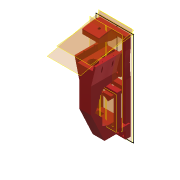
# Autodesk Inventor part: 08_Opentrons_Autofocus_flexurebaering
Saved by Autodesk Inventor 2019.4 (Build 234330000, 330)
## iProperties
Created: 2020-11-20
Part Number: 08_Opentrons_Autofocus_flexurebaering
Material: Generic
Document SubType Name: Modeling
Designer: diederichbenedict
Density: 1 g/cm^3
Appearance: Light Red
Author: diederichbenedict
Autodesk Inventor part; units mm, degrees
ref_plane "YZ Plane" through (0, 0, 0) normal (1, 0, 0) x (0, 1, 0)
ref_plane "XZ Plane" through (0, 0, 0) normal (0, 1, 0) x (-1, 0, 0)
ref_plane "XY Plane" through (0, 0, 0) normal (0, 0, 1) x (1, 0, 0)
ref_plane "Work Plane1" through (0, 0, 0) normal (0, 0, 1) x (1, 0, 0)
sketch "Sketch1" plane through (0, 0, 0) normal (0, 0, 1) x (1, 0, 0)
  line L0 (17.158547, 59.978654) -> (2.158547, 59.978654) construction
  line L1 (2.158547, 59.978654) -> (2.158547, 62.700785) construction
  line L2 (2.158547, 62.700785) -> (17.158547, 62.700785) construction
  line L3 (17.158547, 62.700785) -> (17.158547, 91.339719) construction
  line L4 (6.864659, 91.339719) -> (-18.841453, 91.339719) construction
  line L5 (-18.841453, 91.339719) -> (-18.841453, -14.660281) construction
  line L6 (-18.841453, -14.660281) -> (17.158547, -14.660281) construction
  line L7 (17.158547, -14.660281) -> (17.158547, 59.978654) construction
  line L8 (13.858547, 17.339719) -> (13.863005, 4.639719) construction
  line L9 (13.863005, 4.639719) -> (6.678294, 4.639719) construction
  arc A0 (-15.691453, 17.339719) -> (6.678294, 4.639719) centre (-0.935341, 17.280089) ccw construction
  arc A1 (6.678294, 30.039719) -> (-15.691453, 17.339719) centre (-0.935341, 17.399349) ccw construction
  line L10 (13.863005, 30.039719) -> (6.678294, 30.039719) construction
  line L11 (13.858547, 17.339719) -> (13.863005, 30.039719) construction
  circle A2 centre (-0.935341, 17.399349) radius 10.125
  line L12 (17.158547, -14.660281) -> (-0.935341, -14.660281)
  line L13 (-0.935341, -14.660281) -> (-0.935341, -0.660281)
  line L14 (-0.935341, -0.660281) -> (17.158547, -0.660281)
  line L15 (17.158547, -0.660281) -> (17.158547, -14.660281)
  line L16 (17.158547, 0.876503) -> (13.158547, 0.876503)
  line L17 (13.158547, 0.876503) -> (13.158547, 91.339719)
  line L18 (13.158547, 91.339719) -> (17.158547, 91.339719)
  line L19 (13.158547, 34.280089) -> (-0.935341, 34.280089)
  line L20 (-0.935341, 34.280089) -> (-0.935341, 38.280089)
  line L21 (-0.935341, 38.280089) -> (13.158547, 38.280089)
  line L22 (13.158547, 38.280089) -> (13.158547, 34.280089)
  line L23 (13.158547, 91.339719) -> (-0.935341, 91.339719)
  line L24 (-0.935341, 91.339719) -> (-0.935341, 86.339719)
  line L25 (-0.935341, 86.339719) -> (13.158547, 86.339719)
  line L26 (13.158547, 86.339719) -> (13.158547, 91.339719)
  line L27 (-0.935341, 91.339719) -> (2.064659, 91.339719)
  line L28 (2.064659, 91.339719) -> (2.064659, 103.339719)
  line L29 (2.064659, 103.339719) -> (-0.935341, 103.339719)
  line L30 (-0.935341, 103.339719) -> (-0.935341, 91.339719)
  arc A3 (-5.635247, 28.982133) -> (3.120733, 29.222981) centre (-0.935341, 17.399349) ccw
  arc A4 (-5.635247, 28.982133) -> (3.120733, 29.222981) centre (-0.935341, 17.399349) ccw
  line L31 (14.111603, -3.660281) -> (2.111603, -3.660281) construction
  line L32 (2.111603, -3.660281) -> (2.111603, -11.660281) construction
  line L33 (2.111603, -11.660281) -> (14.111603, -11.660281) construction
  line L34 (14.111603, -11.660281) -> (14.111603, -3.660281) construction
  line L35 (14.111603, -3.660281) -> (2.111603, -11.660281) construction
  line L36 (2.111603, -3.660281) -> (14.111603, -11.660281) construction
  circle A5 centre (14.111603, -3.660281) radius 1.45
  circle A6 centre (14.111603, -11.660281) radius 1.45
  circle A7 centre (2.111603, -3.660281) radius 1.45
  circle A8 centre (2.111603, -11.660281) radius 1.45
  circle A9 centre (-0.935341, 17.399349) radius 10.125
  circle A10 centre (7.722275, -11.660281) radius 1.45
  circle A11 centre (7.722275, -3.660281) radius 1.45
  circle A12 centre (-8.847508, 49.748913) radius 1.45
  circle A13 centre (-9.592957, -3.660281) radius 1.45
  circle A14 centre (7.722275, -3.660281) radius 1.45
  circle A15 centre (14.111603, -11.660281) radius 1.45
  circle A16 centre (7.722275, -11.660281) radius 1.45
  circle A17 centre (-9.592957, -11.660281) radius 1.45
  circle A18 centre (-15.982285, -11.660281) radius 1.45
  circle A19 centre (6.976826, 49.748913) radius 1.45
  line L37 (17.158547, 91.339719) -> (6.864659, 91.339719)
  arc A20 (17.158547, 76.029134) -> (17.158547, 46.231552) centre (138.700705, 61.130343) ccw
  line L38 (17.158547, 91.339719) -> (17.158547, 76.029134)
  line L39 (17.158547, 46.231552) -> (17.158547, 0.876503)
  point P0 (8.111603, -7.660281)
  dimension "d19" = 14
  dimension "d20" = 4
  dimension "d21" = 4
  dimension "d37" = 5
  dimension "d38" = 3
  dimension "d39" = 12
  dimension "d41" = 17
  dimension "d60" = 0
  dimension "d61" = 0
  dimension "d62" = 0
  dimension "d63" = 12
  dimension "d64" = 8
  dimension "d65" = 2.9
  dimension "d66" = 2.9
  dimension "d67" = 2.9
  dimension "d68" = 2.9
  dimension "d83" = 2.9
  dimension "d84" = 2.9
  constraints: 55 end point, 13 parallel, 7 centre point, 6 horizontal, 6 perpendicular, 6 point on line, 4 coincident, 2 midpoint, 2 point on circle
  measures "d19" distance of L12.end L13.end
  measures "d20" distance of L17.end L18.end
  measures "d21" distance of L19.end L20.end
  measures "d37" distance of L24.end L23.end
  measures "d38" distance of L29.end L28.end
  measures "d39" distance of L28.end L27.end
  measures "d41" distance from line of L19 A0.centre
  measures "d60" distance from line of L13 A0.centre
  measures "d61" distance from line of A0.centre L20
  measures "d62" distance from line of A1.centre L24
  measures "d63" distance of L33.end L32.end
  measures "d64" distance of L32.end L31.end
  measures "d65" diameter of A5
  measures "d66" diameter of A6
  measures "d67" diameter of A7
  measures "d68" diameter of A8
  measures "d83" diameter of A10
  measures "d84" diameter of A11
extrude "Extrusion1" add sketch "Sketch1" along normal blind 6 contours L12 L13 L14 L15 | L16 L17 L18 L38 A20 L39 | L19 L20 L21 L17 | L25 L24 L23 L17 | A5 | A7 | A8
ref_plane "Work Plane2" through (0, 0, 11) normal (0, 0, 1) x (1, 0, 0)
sketch "Sketch2" plane through (0, 0, 11) normal (0, 0, 1) x (1, 0, 0)
  line L0 (-0.935341, 34.280089) -> (13.158547, 34.280089)
  line L1 (13.158547, 34.280089) -> (13.158547, 0.876503)
  line L2 (13.158547, 0.876503) -> (17.158547, 0.876503)
  line L3 (17.158547, 76.029134) -> (17.158547, 91.339719) construction
  line L4 (17.158547, 91.339719) -> (-0.935341, 91.339719) construction
  line L5 (13.158547, 86.339719) -> (13.158547, 38.280089) construction
  line L6 (13.158547, 38.280089) -> (-0.935341, 38.280089)
  line L7 (-0.935341, 38.280089) -> (-0.935341, 34.280089)
  line L8 (13.158547, 38.280089) -> (-0.935341, 38.280089)
  line L9 (13.158547, 38.280089) -> (17.158547, 38.280089)
  line L10 (17.158547, 91.339719) -> (-0.935341, 91.339719) construction
  line L11 (13.158547, 91.339719) -> (-0.935341, 91.339719) construction
  line L12 (-0.935341, 91.339719) -> (-0.935341, 86.339719) construction
  line L13 (-0.935341, 86.339719) -> (13.158547, 86.339719) construction
  line L14 (13.158547, 86.339719) -> (13.158547, 91.339719) construction
  line L15 (-0.935341, 91.339719) -> (2.064659, 91.339719) construction
  line L16 (2.064659, 91.339719) -> (2.064659, 99.339719) construction
  line L17 (2.064659, 99.339719) -> (-0.935341, 99.339719) construction
  line L18 (-0.935341, 99.339719) -> (-0.935341, 91.339719) construction
  line L19 (-0.935341, 91.339719) -> (-0.935341, 86.339719) construction
  line L20 (-0.935341, 86.339719) -> (13.158547, 86.339719) construction
  line L21 (17.158547, 0.876503) -> (17.158547, 46.231552)
  arc A0 (17.158547, 76.029134) -> (17.158547, 46.231552) centre (138.700705, 61.130343) ccw construction
  line L22 (-0.935341, 38.280089) -> (13.158547, 38.280089)
  line L23 (-0.935341, 38.280089) -> (17.158547, 38.280089)
  line L24 (17.158547, 38.280089) -> (17.158547, 34.280089)
  line L25 (17.158547, 34.280089) -> (-0.935341, 34.280089)
  line L26 (-0.935341, 34.280089) -> (-0.935341, 38.280089)
  line L27 (13.158547, 0.876503) -> (17.158547, 0.876503)
  line L28 (17.158547, 34.280089) -> (13.158547, 34.280089)
  line L29 (13.158547, 34.280089) -> (13.158547, 0.876503)
  line L30 (13.158547, 0.876503) -> (17.158547, 0.876503)
  line L31 (17.158547, 0.876503) -> (17.158547, 34.280089)
  point P0 (0, 0)
  point P1 (2.064659, 91.339719)
  dimension "d34" = 5
  dimension "d35" = 3
  dimension "d36" = 8
  constraints: 34 end point, 8 parallel, 5 perpendicular, 4 horizontal, 2 point on line
  measures "d34" distance of L12.end L10.end
  measures "d35" distance of L17.end L16.end
  measures "d36" distance of L16.end L15.end
extrude "Extrusion2" add sketch "Sketch2" along normal blind 5
sketch "Sketch3" plane through (17.158547, -14.660281, 0) normal (1, 0, 0) x (0, 0, -1)
  line L0 (0, 14) -> (0, 0)
  line L1 (0, 14) -> (-6, 14)
  line L2 (-6, 0) -> (-6, 14)
  line L3 (0, 0) -> (-6, 0)
  line L4 (0, 90.689414) -> (0, 106)
  line L5 (0, 106) -> (-6, 106)
  line L6 (-6, 90.689414) -> (-6, 106)
  line L7 (-11, 106) -> (-11, 94.797626)
  line L8 (-16, 94.797626) -> (-16, 106)
  line L9 (-6, 14) -> (-6, 0)
  line L10 (-11.5, 14.036784) -> (-6, 14.036784)
  line L11 (-6, 14.036784) -> (-6, 9.036784)
  line L12 (-6, 9.036784) -> (-11.5, 9.036784)
  line L13 (-11.5, 9.036784) -> (-11.5, 14.036784)
  line L14 (-11, 15.536784) -> (-16, 15.536784)
  line L15 (-11, 15.536784) -> (-11.5, 15.536784)
  line L16 (-11.5, 15.536784) -> (-11.5, 14.036784)
  line L17 (-11.5, 14.036784) -> (-11, 14.036784)
  line L18 (-11, 14.036784) -> (-11, 15.536784)
  line L19 (0, 15.536784) -> (-0.5, 15.536784)
  line L20 (-0.5, 15.536784) -> (-0.5, 14)
  line L21 (-0.5, 14) -> (0, 14)
  line L22 (0, 14) -> (0, 15.536784)
  line L23 (-6, 15.536784) -> (-6, 106)
  line L24 (-6, 54.44037) -> (-11.5, 54.44037)
  line L25 (-11.5, 54.44037) -> (-11.5, 59.44037)
  line L26 (-11.5, 59.44037) -> (-6, 59.44037)
  line L27 (-6, 59.44037) -> (-6, 54.44037)
  line L28 (-11, 52.94037) -> (-16, 52.94037)
  line L29 (-11, 52.94037) -> (-11.5, 52.94037)
  line L30 (-11.5, 52.94037) -> (-11.5, 54.44037)
  line L31 (-11.5, 54.44037) -> (-11, 54.44037)
  line L32 (-11, 54.44037) -> (-11, 52.94037)
  line L33 (0, 90.689414) -> (-6, 90.689414)
  line L34 (-11, 106) -> (-16, 106)
  line L35 (-11, 94.797626) -> (-16, 94.797626)
  point P0 (0, 14.660281)
  dimension "d25" = 5
  dimension "d26" = 0.5
  dimension "d27" = 0.5
  dimension "d28" = 5
  dimension "d29" = 0.5
  dimension "d40" = 0
  constraints: 40 end point, 10 parallel, 6 point on line, 5 horizontal, 5 perpendicular
  measures "d25" distance of L10.end L11.end
  measures "d26" distance of L17.end L16.end
  measures "d27" distance of L21.end L20.end
  measures "d28" distance of L24.end L25.end
  measures "d29" distance of L30.end L31.end
  measures "d40" distance between parallel lines of L30 L25
extrude "Extrusion3" add sketch "Sketch3" against normal up to surface (4 mm away) contours L1 L20 L19 L22 | L2 L12 L13 L10 L11 | L10 L16 L14 L18
ref_plane "Work Plane3" through (0, 0, 18) normal (0, 0, 1) x (1, 0, 0)
sketch "Sketch4" plane through (0, 0, 18) normal (0, 0, 1) x (1, 0, 0)
  line L0 (17.158547, 34.889127) -> (-18.841453, 34.889127)
  line L1 (-0.935341, 34.280089) -> (13.158547, 34.280089)
  line L2 (13.158547, 34.280089) -> (13.158547, 0.876503)
  line L3 (13.158547, 0.876503) -> (17.158547, 0.876503)
  line L4 (-0.935341, 38.280089) -> (-0.935341, 34.280089)
  line L5 (-4.526541, 27.364099) -> (2.655859, 27.364099)
  arc A0 (9.489986, 15.527045) -> (2.655859, 27.364099) centre (-0.935341, 17.399349) ccw
  line L6 (9.489986, 15.527045) -> (5.898786, 9.306903)
  arc A1 (-7.769468, 9.306903) -> (5.898786, 9.306903) centre (-0.935341, 17.399349) ccw
  line L7 (-7.769468, 9.306903) -> (-11.360668, 15.527045)
  arc A2 (-4.526541, 27.364099) -> (-11.360668, 15.527045) centre (-0.935341, 17.399349) ccw
  arc A3 (-3.214574, 30.399349) -> (-4.800903, 29.617364) centre (-3.214574, 28.399349) ccw
  arc A4 (-5.635247, 28.982133) -> (-4.800903, 29.617364) centre (-6.387232, 30.835378) ccw
  arc A5 (-5.635247, 28.982133) -> (3.120733, 29.222981) centre (-0.935341, 17.399349) ccw
  arc A6 (2.301156, 29.757056) -> (3.120733, 29.222981) centre (3.769704, 31.114762) ccw
  arc A7 (2.301156, 29.757056) -> (0.832608, 30.399349) centre (0.832608, 28.399349) ccw
  line L8 (0.832608, 30.399349) -> (-3.214574, 30.399349)
  arc A8 (2.411297, 29.858883) -> (0.832608, 30.549349) centre (0.832608, 28.399349) ccw
  arc A9 (2.411297, 29.858883) -> (3.169405, 29.364864) centre (3.769704, 31.114762) ccw
  arc A10 (-5.691646, 29.121126) -> (3.169405, 29.364864) centre (-0.935341, 17.399349) ccw
  arc A11 (-5.691646, 29.121126) -> (-4.919877, 29.708715) centre (-6.387232, 30.835378) ccw
  arc A12 (-3.214574, 30.549349) -> (-4.919877, 29.708715) centre (-3.214574, 28.399349) ccw
  line L9 (-3.214574, 30.549349) -> (0.832608, 30.549349)
  line L10 (8.265033, 26.081262) -> (11.868953, 29.685181)
  line L11 (8.265033, 26.081262) -> (13.361745, 26.081262) construction
  line L12 (11.868953, 29.685181) -> (11.868953, 32.780089)
  line L13 (11.868953, 32.780089) -> (-0.935341, 32.780089)
  line L14 (-0.935341, 38.280089) -> (-0.935341, 34.280089)
  line L15 (-0.935341, 33.557251) -> (-0.935341, 30.549349)
  line L16 (-0.935341, 32.780089) -> (-0.935341, 30.549349)
  line L17 (17.158547, 0.876503) -> (17.158547, 38.280089) construction
  line L18 (17.158547, 0.876503) -> (17.158547, 38.280089)
  line L19 (17.158547, 0.876503) -> (17.158547, 34.889127)
  line L20 (17.158547, 38.280089) -> (-0.935341, 38.280089)
  point P0 (0, 0)
  point P1 (17.158547, 49.748913)
  dimension "d43" = 0.15
  dimension "d44" = 45
  dimension "d49" = 1.5
  constraints: 18 end point, 11 point on circle, 5 centre point, 4 point on line, 2 horizontal, 2 vertical, 1 collinear, 1 equal length, 1 perpendicular, 7 other
  measures "d43" radial gap between concentric circles of A7 A8
  measures "d44" angle of L11 L10
  measures "d49" distance between parallel lines of L1 L13
extrude "Extrusion4" add sketch "Sketch4" against normal up to surface (18 mm away) contours A8 L9 L15 L13 L12 L10 A10 A9
sketch "Sketch5" plane through (-0.935341, 30.549349, 18) normal (-1, 0, 0) x (0, 0, 1)
  line L0 (-7, 3.73074) -> (-7, 7.73074)
  line L1 (-7, 3.73074) -> (-2, 3.73074)
  line L2 (-2, 7.73074) -> (-2, 3.73074)
  line L3 (-7, 7.73074) -> (-2, 7.73074)
  line L4 (-18, 0) -> (-18, 2.23074)
  line L5 (0, 0) -> (-18, 0)
  line L6 (0, 2.23074) -> (0, 0)
  line L7 (0, 2.23074) -> (-18, 2.23074)
  line L8 (-18, 3.73074) -> (-18, 7.73074)
  line L9 (-18, 3.73074) -> (-12, 3.73074)
  line L10 (-12, 7.73074) -> (-12, 3.73074)
  line L11 (-18, 7.73074) -> (-12, 7.73074)
  line L12 (0, 2.23074) -> (-18, 2.23074)
  line L13 (-18, 3.73074) -> (-17.5, 3.73074)
  line L14 (-17.5, 3.73074) -> (-17.5, 2.23074)
  line L15 (-17.5, 2.23074) -> (-18, 2.23074)
  line L16 (-18, 2.23074) -> (-18, 3.73074)
  line L17 (-7, 3.73074) -> (-6.5, 3.73074)
  line L18 (-6.5, 3.73074) -> (-6.5, 2.23074)
  line L19 (-6.5, 2.23074) -> (-7, 2.23074)
  line L20 (-7, 2.23074) -> (-7, 3.73074)
  point P0 (-18, -30.549349)
  dimension "d47" = 0.5
  dimension "d48" = 0.5
  constraints: 16 end point, 4 parallel, 2 horizontal, 2 perpendicular, 2 point on line
  measures "d47" distance of L14.end L15.end
  measures "d48" distance of L18.end L19.end
sketch "Sketch7" plane through (-0.935341, 32.780089, 18) normal (0, 1, 0) x (1, 0, 0)
  circle A0 centre (-0.255642, 2.740799) radius 1.45
  line L0 (-0.255642, 2.740799) -> (-0.255642, 18) construction
  line L1 (1.394358, 2.740799) -> (1.394358, 18)
  line L2 (-1.905642, 18) -> (-1.905642, 2.740799)
  arc A1 (-1.905642, 2.740799) -> (1.394358, 2.740799) centre (-0.255642, 2.740799) ccw
  arc A2 (1.394358, 18) -> (-1.905642, 18) centre (-0.255642, 18) ccw
  line L3 (-0.255642, 2.740799) -> (15.003559, 2.740799) construction
  point P0 (0.935341, 18)
  point P1 (-0.255642, 10.370399)
  dimension "d50" = 90
  dimension "d51" = 0.2
  constraints: 10 end point, 4 point on circle, 4 tangent, 2 centre point, 1 horizontal, 1 midpoint, 1 parallel, 1 perpendicular
  measures "d50" angle of L3 L0
  measures "d51" radial gap between concentric circles of A0 A1
extrude "Extrusion5" cut sketch "Sketch7" against normal blind 5 contours A0 | A1 L2 A2 L1
extrude "Extrusion6" add sketch "Sketch5" against normal up to surface (12.804294 mm away) contours L1 L18 L7 L20 | L7 L16 L9 L14
sketch "Sketch8" plane through (0, 0, 18) normal (0, 0, 1) x (1, 0, 0)
  arc A0 (2.411297, 29.858883) -> (0.832608, 30.549349) centre (0.832608, 28.399349) ccw
  arc A1 (2.411297, 29.858883) -> (3.169405, 29.364864) centre (3.769704, 31.114762) ccw
  arc A2 (8.265033, 26.081262) -> (3.169405, 29.364864) centre (-0.935341, 17.399349) ccw
  line L0 (8.265033, 26.081262) -> (11.868953, 29.685181)
  line L1 (11.868953, 29.685181) -> (11.868953, 32.780089)
  line L2 (11.868953, 32.780089) -> (-0.935341, 32.780089)
  line L3 (-0.935341, 32.780089) -> (-0.935341, 30.549349)
  line L4 (-0.935341, 30.549349) -> (0.832608, 30.549349)
  line L5 (11.868953, 34.280089) -> (11.868953, 32.780089)
  line L6 (-0.935341, 34.280089) -> (11.868953, 34.280089)
  line L7 (-0.935341, 32.780089) -> (-0.935341, 34.280089)
  line L8 (-0.935341, 32.780089) -> (0.459017, 32.780089)
  line L9 (11.868953, 32.780089) -> (0.459017, 32.780089)
  line L10 (-0.895411, 34.280089) -> (2.604589, 34.280089)
  line L11 (2.604589, 34.280089) -> (2.604589, 31.780089)
  line L12 (2.604589, 31.780089) -> (-0.895411, 31.780089)
  line L13 (-0.895411, 31.780089) -> (-0.895411, 34.280089)
  point P0 (0, 0)
  dimension "d56" = 3.5
  dimension "d57" = 2.5
  constraints: 8 end point, 2 parallel, 1 horizontal, 1 perpendicular, 1 point on line
  measures "d56" distance of L11.end L12.end
  measures "d57" distance of L10.end L11.end
extrude "Extrusion7" cut sketch "Sketch8" against normal through all contours L13 L6 L11 L2 | L2 L11 L12 L13
sketch "Sketch9" plane through (-0.935341, -14.660281, 0) normal (-1, 0, 0) x (0, 0, 1)
  line L0 (0, 0) -> (0, 14)
  line L1 (0, 0) -> (6, 0)
  line L2 (6, 14) -> (6, 0)
  line L3 (0, 14) -> (6, 14)
  line L4 (24.051888, 27.109882) -> (31.122956, 34.18095)
  line L5 (29.708742, 35.595164) -> (22.637674, 28.524096)
  line L6 (31.122956, 34.18095) -> (29.708742, 35.595164)
  line L7 (24.051888, 27.109882) -> (22.637674, 28.524096)
  line L8 (29.708742, 35.736585) -> (22.496253, 28.524096)
  line L9 (24.051888, 26.968461) -> (31.264377, 34.18095)
  line L10 (31.264377, 34.18095) -> (29.708742, 35.736585)
  line L11 (22.496253, 28.524096) -> (38.52182, 28.524096) construction
  line L12 (0, 14) -> (6, 14)
  line L13 (15.723556, 14) -> (6, 14)
  line L14 (6, 14) -> (6, 0)
  line L15 (29.708742, 35.736585) -> (29.708742, 57.736585)
  line L16 (29.708742, 57.736585) -> (0, 57.736585)
  line L17 (0, 101) -> (0, 52.94037)
  line L18 (0, 57.736585) -> (0, 63.736585)
  line L19 (0, 63.736585) -> (35.708742, 63.736585)
  line L20 (35.708742, 63.736585) -> (35.708742, 34.18095)
  line L21 (35.708742, 34.18095) -> (19.769903, 0)
  line L22 (0, 0) -> (6, 0)
  line L23 (19.769903, 0) -> (6, 0)
  line L24 (0, 57.736585) -> (22.116428, 54.292028)
  line L25 (22.116428, 54.292028) -> (29.708742, 35.736585)
  line L26 (15.723556, 14) -> (22.496253, 16.430232)
  line L27 (22.496253, 16.430232) -> (22.496253, 25.412826)
  line L28 (22.496253, 28.524096) -> (22.372688, 28.259109)
  line L29 (19.901381, 22.959376) -> (19.777816, 22.694389)
  line L30 (24.051888, 26.968461) -> (22.496253, 25.412826)
  line L31 (22.496253, 28.524096) -> (22.566964, 28.453385)
  line L32 (23.981177, 27.039172) -> (24.051888, 26.968461)
  point P0 (0, 14.660281)
  dimension "d69" = 0.1
  dimension "d71" = 22
  dimension "d72" = 6
  dimension "d73" = 6
  constraints: 48 end point, 7 point on line, 4 perpendicular, 3 parallel, 2 vertical, 1 collinear, 1 horizontal, 3 other
  measures "d69" distance between parallel lines of L6 L10
  measures "d71" distance of L8.start L15.end
  measures "d72" distance of L16.end L18.end
  measures "d73" distance between parallel lines of L20 L15
extrude "Extrusion8" add sketch "Sketch9" against normal blind 7 contours L2 L13 L26 L27 L30 L9 L10 L15 L16 L17 L19 L20 L21 L23 | L16 L15 L25 L24
sketch "Sketch10" plane through (-0.935341, 19.520669, 35.708742) normal (0, 0, 1) x (1, 0, 0)
  line L0 (12.5, 51.984385) -> (-12.5, 51.984385)
  line L1 (0, 29.555635) -> (7, 29.555635)
  line L2 (12.5, 51.984385) -> (7, 29.555635)
  line L3 (0, 29.555635) -> (7, 29.555635)
  line L4 (0, 29.555635) -> (0, 46.163435)
  line L5 (0, 46.163435) -> (8.895627, 46.163435)
  line L6 (8.895627, 46.163435) -> (10.323046, 51.984385)
  line L7 (12.5, 51.984385) -> (10.323046, 51.984385)
  point P0 (0.935341, -19.520669)
  constraints: 10 end point, 2 parallel, 1 perpendicular, 1 point on line, 1 vertical
extrude "Extrusion9" add sketch "Sketch10" against normal up to surface (35.708742 mm away)
sketch "Sketch11" plane through (9.387705, 71.505055, 35.708742) normal (0, 1, 0) x (1, 0, 0)
  circle A0 centre (0.176954, 22.035534) radius 1.05
  circle A1 centre (0.176954, 9.535534) radius 1.05
  ellipse E0 centre (-10.323046, 9.535534) end of major axis (-12.255236, 9.535534) minor radius 1.366265
  circle A2 centre (-10.323046, 9.535534) radius 5
  circle A3 centre (0.176954, 22.035534) radius 0.95
  circle A4 centre (0.176954, 9.535534) radius 0.95
  line L0 (-10.323046, 18.863419) -> (-10.323046, 34.929483) construction
  line L1 (-8.873046, 20.313419) -> (-8.873046, 33.479483)
  line L2 (-11.773046, 33.479483) -> (-11.773046, 20.313419)
  arc A5 (-11.773046, 20.313419) -> (-8.873046, 20.313419) centre (-10.323046, 20.313419) ccw
  arc A6 (-8.873046, 33.479483) -> (-11.773046, 33.479483) centre (-10.323046, 33.479483) ccw
  arc A7 (-10.283116, 18.82623) -> (-8.928688, 20.449541) centre (-10.578688, 20.449541) ccw
  point P0 (-9.387705, 35.708742)
  point P1 (-10.323046, 26.896451)
  point P2 (-10.323046, 35.208742)
  dimension "d78" = 10
  dimension "d79" = 1.9
  dimension "d80" = 1.9
  dimension "d99" = 2.9
  constraints: 8 end point, 6 point on circle, 5 centre point, 4 tangent, 3 coincident, 2 point on line, 1 midpoint, 1 parallel, 1 vertical, 1 other
  measures "d78" diameter of A2
  measures "d79" diameter of A3
  measures "d80" diameter of A4
  measures "d99" diameter of A6
extrude "Extrusion10" cut sketch "Sketch11" against normal up to surface (33.224965 mm away) contours E0 | A2 | A3 | A4 | A5 L2 A6 L1
sketch "Sketch12" plane through (0, 0, 6) normal (0, 0, 1) x (1, 0, 0)
  line L0 (-0.935341, 19.520669) -> (-0.935341, 65.684104)
  line L1 (-0.935341, 19.520669) -> (6.064659, 19.520669)
  line L2 (6.064659, 49.076304) -> (6.064659, 19.520669)
  line L3 (6.064659, 49.076304) -> (11.564659, 71.505055)
  line L4 (11.564659, 71.505055) -> (9.387705, 71.505055)
  line L5 (9.387705, 71.505055) -> (7.960286, 65.684104)
  line L6 (7.960286, 65.684104) -> (-0.935341, 65.684104)
  line L7 (6.064659, 43.076304) -> (6.064659, 49.076304)
  line L8 (6.064659, 46.076304) -> (11.064659, 46.076304)
  line L9 (11.064659, 46.076304) -> (11.064659, 69.466078)
  circle A0 centre (6.976826, 49.748913) radius 1.45
  point P0 (0, 0)
  dimension "d85" = 5
  dimension "d86" = 2.9
  constraints: 4 end point, 1 centre point, 1 horizontal, 1 midpoint, 1 perpendicular, 1 point on line
  measures "d85" distance of L8.start L8.end
  measures "d86" diameter of A0
extrude "Extrusion11" add sketch "Sketch12" against normal up to surface (6 mm away) contours L2 A0 L3 L9 L8
mirror "Mirror2" about plane through (-0.935341, -0.660281, 0) normal (-1, 0, 0) of "Extrusion1", "Extrusion2", "Extrusion3", "Extrusion4", "Extrusion5", "Extrusion6", "Extrusion7", "Extrusion8", "Extrusion9", "Extrusion10", "Extrusion11"
sketch "Sketch19" plane through (-19.029229, 76.029134, 0) normal (-1, 0, 0) x (0, 0, 1)
  line L0 (0, 0) -> (0, 15.310586)
  line L1 (0, 0) -> (6, 0)
  line L2 (6, 0) -> (6, 15.310586)
  line L3 (0, 15.310586) -> (6, 15.310586)
  line L4 (6, 0) -> (6, 15.310586)
  line L5 (6, 14.675797) -> (0, 14.077822)
  line L6 (0, 0) -> (0, 15.310586)
  line L7 (0, 15.310586) -> (6, 15.310586)
  line L8 (0, 15.310586) -> (6, 15.310586)
  line L9 (6, 15.310586) -> (6, 14.675797)
  point P0 (0, -76.029134)
  constraints: 6 end point, 2 point on line, 1 horizontal, 1 perpendicular
extrude "Extrusion18" cut sketch "Sketch19" against normal through all contours L0 L3 L2 L5
sketch "Sketch22" plane through (-19.029229, 76.029134, 0) normal (-1, 0, 0) x (0, 0, 1)
  line L0 (0.5, -75.152631) -> (6, -75.152631)
  line L1 (0, 14.077822) -> (6, 14.675797)
  circle A0 centre (0.5, -75.152631) radius 89.996647
  line L2 (21.131123, 12.447331) -> (21.131123, 7.147654)
  line L3 (21.131123, 7.147654) -> (6, 2.763748)
  line L4 (6, 2.763748) -> (6, 14.675797)
  line L5 (6, 2.763748) -> (0, 2.763748)
  line L6 (0, 2.763748) -> (0, 14.842627)
  line L7 (0, 14.842627) -> (6, 14.842627)
  line L8 (6, 14.842627) -> (6, 2.763748)
  point P0 (0, -76.029134)
  constraints: 14 end point, 3 parallel, 3 point on circle, 1 centre point, 1 coincident, 1 horizontal, 1 perpendicular, 1 point on line, 1 vertical
sketch "Sketch22 outline for Extrusion21" plane through (-19.029229, 76.029134, 0) normal (-1, 0, 0) x (0, 0, 1)
  line L0 (0, 2.763748) -> (6, 2.763748)
  line L1 (6, 2.763748) -> (21.131123, 7.147654)
  line L2 (21.131123, 7.147654) -> (21.131123, 12.447331)
  arc A0 (21.131123, 12.447331) -> (6, 14.675797) centre (0.5, -75.152631) ccw
  line L3 (6, 14.675797) -> (0, 14.077822)
  line L4 (0, 14.077822) -> (0, 2.763748)
extrude "Extrusion21" add sketch "Sketch22 outline for Extrusion21" against normal blind 20
ref_plane "Work Plane10" through (-19.029229, 86.339719, 30.203764) normal (0, 0.99332, 0.1153924) x (-1, 0, 0)
ref_plane "Work Plane9" through (-19.029229, 88.476464, 21.131123) normal (0, 0.9733692, 0.2292432) x (-1, 0, 0)
sketch "Sketch23" plane through (-19.029229, 86.339719, 30.203764) normal (0, 0.99332, 0.1153924) x (-1, 0, 0)
  line L0 (-8.958069, -2.707135) -> (-8.958069, -20.303467)
  line L1 (-14.158069, -2.707135) -> (-14.158069, -20.303467)
  line L2 (-32.187776, -18.034795) -> (-4, -18.034795)
  circle A0 centre (-11.558069, -18.034795) radius 1.45
  point P0 (-19.029229, -20.039051)
  dimension "d121" = 2.9
  dimension "d122" = 2.6
  constraints: 4 end point, 2 vertical, 1 centre point, 1 point on line, 4 other
  measures "d121" diameter of A0
  measures "d122" distance from line of A0.centre L0
extrude "Extrusion22" cut sketch "Sketch23" along normal mid plane 20
sketch "Sketch24" plane through (0, 0, 0) normal (0, 0, -1) x (-1, 0, 0)
  line L0 (-0.970771, 78.792882) -> (-0.970771, 86.339719)
  line L1 (-20.556352, -19.461789) -> (-0.970771, -19.461789)
  line L2 (-0.970771, -19.461789) -> (-0.970771, 91.647864)
  line L3 (-0.970771, 91.647864) -> (-20.556352, 91.647864)
  line L4 (-20.556352, 91.647864) -> (-20.556352, -19.461789)
  line L5 (23.977023, -18.958271) -> (-0.970771, -18.958271)
  line L6 (-0.970771, -18.958271) -> (-0.970771, 78.792882)
  line L7 (-0.970771, 78.792882) -> (23.977023, 78.792882)
  line L8 (23.977023, 78.792882) -> (23.977023, -18.958271)
  line L9 (-13.158547, 86.339719) -> (-0.970771, 86.339719)
  line L10 (23.977023, 78.792882) -> (14.903296, 78.792882)
  line L11 (14.903296, 78.792882) -> (14.903296, 86.511969)
  line L12 (14.903296, 86.511969) -> (23.977023, 86.511969)
  line L13 (23.977023, 86.511969) -> (23.977023, 78.792882)
  line L14 (23.977023, 86.511969) -> (-0.970771, 86.511969)
  line L15 (-0.970771, 86.511969) -> (-0.970771, 91.647864)
  line L16 (-0.970771, 91.647864) -> (23.977023, 91.647864)
  line L17 (23.977023, 91.647864) -> (23.977023, 86.511969)
  point P0 (0, 0)
  constraints: 32 end point, 8 parallel, 4 horizontal, 4 perpendicular
ref_plane "Work Plane6" through (-1.870682, 0, 11) normal (0, 0, -1) x (-1, 0, 0)
ref_plane "Work Plane7" through (-1.870682, 0, 18) normal (0, 0, -1) x (-1, 0, 0)
body "Solid1"
